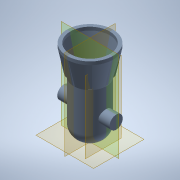
# Autodesk Inventor part: Waterkanon
Saved by Autodesk Inventor 2021 (Build 250183000, 183)
## iProperties
Manager: Pierloot J.
Company: Emmaüs Bovenbouw Aalter
Created: 2015-08-18
Part Number: Waterkanon
Material: S235
Catalog Web Link: http://emmausbovenbouw.op-weg.be/
Vendor: Emmaüsinstituut Bovenbouw Aalter
Document SubType Name: Modeling
Designer: Pierlootj
Engineer: Pierloot J.
Manufacturer: Standard
Standards Organization: Custom
Density: 7.86 g/cm^3
Appearance: Light Steel Blue
Title: Algemene titel
Subject: Specifieke titel
Author: Pierlootj
Keywords: Ruwe Ø xxxxx
Comments: Opmerking
Autodesk Inventor part; units mm, degrees
sketch "Sketch19" plane through (0, 0, 0) normal (0, 0, 1) x (1, 0, 0)
  circle A0 centre (0, 0) radius 12.5
  dimension "d130" = 25
  constraints: 1 centre point, 1 coincident
  measures "d130" diameter of A0
extrude "Extrusion17" add sketch "Sketch19" along normal blind 40
sketch "Sketch20" plane through (0, 0, 40) normal (0, 0, 1) x (1, 0, 0)
  circle A0 centre (0, 0) radius 10
  dimension "d133" = 20
  constraints: 1 centre point, 1 coincident
  measures "d133" diameter of A0
fillet "Fillet6" radius 10 1 edges at (-12.5, 0, 0)
extrude "Extrusion18" cut sketch "Sketch20" against normal blind 25
ref_plane "Work Plane3" through (10, 0, 0) normal (1, 0, 0) x (0, 1, 0)
sketch "Sketch21" plane through (10, 0, 0) normal (1, 0, 0) x (0, 1, 0)
  line L0 (0, 0) -> (0, 20)
  circle A0 centre (0, 20) radius 5
  dimension "d138" = 20
  dimension "d139" = 10
  constraints: 2 end point, 1 centre point, 1 coincident, 1 vertical
  measures "d138" distance of L0.start L0.end
  measures "d139" diameter of A0
extrude "Extrusion19" add sketch "Sketch21" along normal blind 10
mirror "Mirror1" about plane through (0, 0, 0) normal (1, 0, 0) of "Extrusion19"
sketch "Sketch22" plane through (-20, 0, 20) normal (-1, 0, 0) x (0, 0, 1)
  circle A0 centre (0, 0) radius 2.5
  point P0 (-20, 0)
  dimension "d142" = 5
  constraints: 1 centre point
  measures "d142" diameter of A0
extrude "Extrusion20" cut sketch "Sketch22" against normal blind 3
sketch "Sketch26" plane through (0, 0, 0) normal (1, 0, 0) x (0, 1, 0)
  line L0 (-10, 40) -> (10, 40) projected
  line L1 (12.5, 40) -> (-12.5, 40) projected
  line L2 (10, 40) -> (12.5, 40)
  line L3 (17.5, 60) -> (12.5, 40)
  line L4 (17.5, 60) -> (17.5, 62.5)
  line L5 (17.5, 62.5) -> (15, 62.5)
  line L6 (15, 62.5) -> (15, 60)
  line L7 (10, 40) -> (15, 60)
  line L8 (0, -10.5) -> (0, 63) projected
  point P0 (0, 0)
  dimension "d147" = 2.5
  dimension "d148" = 2.5
  constraints: 12 end point, 1 horizontal, 1 perpendicular, 1 vertical
  measures "d147" distance of L3.start L4.end
  measures "d148" distance of L4.end L5.end
revolve "Revolution1" add sketch "Sketch26" angle 360 about axis through (0, 0, -10) along (0, 0, 1)
sketch "Sketch27" plane through (0, 0, 0) normal (1, 0, 0) x (0, 1, 0)
  line L0 (12.5, 40) -> (13.7856, 41.5321)
  line L1 (12.5, 40) -> (14.5, 40) construction
  line L2 (13.7856, 41.5321) -> (17.5, 60)
  line L3 (12.5, 40) -> (-12.5, 40) projected
  line L4 (12.5, 40) -> (11.5, 40)
  line L5 (-17.5, 60) -> (17.5, 60) projected
  line L6 (17.5, 60) -> (16.5, 60)
  line L7 (16.5, 60) -> (11.5, 40)
  point P0 (0, 0)
  dimension "d150" = 2
  dimension "d151" = 50
  dimension "d152" = 1
  dimension "d153" = 1
  constraints: 12 end point, 2 point on line, 1 equal length, 1 horizontal
  measures "d150" distance of L0.start L0.end
  measures "d151" angle of L1 L0
  measures "d152" distance of L0.start L4.end
  measures "d153" distance of L2.end L6.end
extrude "Extrusion21" add sketch "Sketch27" along normal mid plane 2
pattern_circular "Circular Pattern2" count 8 over 360 about axis through (0, 0, -10) along (0, 0, 1) of "Extrusion21"
body "Solid8"
